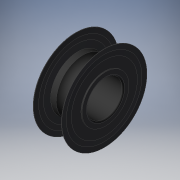
# Autodesk Inventor part: SKF_608-2RSL_PART1
Saved by Autodesk Inventor 2019 (Build 230136000, 136)
## iProperties
Created: 2022-07-08
Part Number: SKF_608-2RSL_PART1
Material: Generic
Catalog Web Link: www.cadenas.de
Description: -Deep groove ball bearings
Vendor: SKF
Document SubType Name: Modeling
Designer: psAdmin
Manufacturer: SKF
Mass: 12 g
Surface Area: 13.7399 cm^2
Volume: 0.419446 cm^3
Density: 1 g/cm^3
Appearance: PSOLRGB-175-175-175
Category: PARTsolutions
Company: SKF
Title: SKF_608-2RSL_PART1
Author: Cadenas PARTsolutions
Comments: Deep groove ball bearings
PSOL_IDENT_0: {$CADENAS_DATA/23d-libs/skf/bearings_units_and_housings/ball_bearings/deep_groove_ball_bearings/bb1_
PSOL_IDENT_1: 001_101.prj},202 {VTYP=3D},{NB=SKF_608-2RSL_PART1},{LINA=SKF_608-2RSL_PART1},{NN=BB1_001_101_PART1},
PSOL_IDENT_2: {NOPRJ=TRUE},{DATE=08.07.2022 10:24:27},{GEOMDATE=04.07.2022 10:54:51},{VERSION=},{LINEID=7700},{WBV
PSOL_IDENT_3: AR=},{WBNUMERIC=}  {NB=SKF_608-2RSL_PART1},{LINA=SKF_608-2RSL_PART1},{KT=DUMMY},{DESIGNATION=608-2RS
PSOL_IDENT_4: L},{R12=0.30},{DD=8.000},{D=22.000},{B=7.000},{C=},{CX=},{CXX=},{CA=0.000},{XXVARIANT=},{XXDESIGN=Si
PSOL_IDENT_5: ngle row},{XXSEALING=Low-friction seal on both sides},{DESIGN=dgbb2rs},{DESIGNIR=dgbb2rs},{VARIANT=}
PSOL_IDENT_6: ,{DD1=12.15},{DD2=10.55},{DD2X=},{DD2A=10.55},{D1=17.60},{D1X=0.00},{D2=19.2},{D2A=19.20},{D3=},{D3X=
PSOL_IDENT_7: },{D3A=0.000},{D4=},{HH=0.000},{BB=0.000},{BBX=},{BBA=0.000},{FF=},{R0MAX=0.000},{R0=0.000},{PITCH=1
PSOL_IDENT_8: 4.70},{DW=3.969},{DDAMIN=10.000},{DDAMAX=10.500},{DDBMIN=0.000},{DDBMAX=0.000},{DBMIN=0.000},{DAMAX=
PSOL_IDENT_9: 20.000},{BBAMIN=0.000},{CAMAX=0.000},{RAMAX=0.300},{LOAD1=3.450},{LOAD2=1.370},{LOAD3=0.057},{SPEED1=
PSOL_IDENT_10: 75000},{SPEED2=38000},{KR=0.025},{F0=12.000},{Z=7},{II=1},{MASS=0.012},{BEARING=608-2RSL},{RING=},{H
PSOL_IDENT_11: ELP=2.200},{HELP2=1.400},{DD1ALG=6.075},{YALG=6.075},{PITCH1=14.700},{DW1=3.969},{YALG1=8.800},{HALG
PSOL_IDENT_12: 1=2.200},{SH=5.275},{CU=0.606},{HALG=2.075},{B1=0},{SHIELDHELP=2},{D4A=0.000},{FFA=0.000},{RS1=},{HE
PSOL_IDENT_13: LP3=0}
NB: SKF_608-2RSL_PART1
NT: Deep groove ball bearings
NBSYN: SKF_$DESIGNATION._PART1
LINA: SKF_608-2RSL_PART1
CATALOG: SKF
DESIGNATION: 608-2RSL
R12: 0.3
DD: 8
D: 22
B: 7
XXDESIGN: Single row
XXSEALING: Low-friction seal on both sides
DD2: 10.55
D2: 19.2
LOAD1: 3.45
LOAD2: 1.37
LOAD3: 0.057
SPEED1: 75000
SPEED2: 38000
BEARING: 608-2RSL
SUPPLIER: SKF
ARTICLENO: SKF_608-2RSL_PART1
BOMINFO: SKF_608-2RSL_PART1
CREATOR: CADENAS GmbH
Autodesk Inventor part; units mm, degrees
ref_plane "YZ Plane" through (0, 0, 0) normal (1, 0, 0) x (0, 1, 0)
ref_plane "XZ Plane" through (0, 0, 0) normal (0, 1, 0) x (-1, 0, 0)
ref_plane "XY Plane" through (0, 0, 0) normal (0, 0, 1) x (1, 0, 0)
sketch "Sketch_58" plane through (0, 0, 0) normal (0, 0, 1) x (1, 0, 0)
  line L0 (50, 0) -> (-50, 0)
  line L1 (0, 5.975) -> (0, 4.3)
  arc A0 (0, 4.3) -> (0.3, 4) centre (0.3, 4.3) ccw
  line L2 (0.3, 4) -> (6.7, 4)
  arc A1 (6.7, 4) -> (7, 4.3) centre (6.7, 4.3) ccw
  line L3 (7, 4.3) -> (7, 5.975)
  arc A2 (7, 5.975) -> (6.9, 6.075) centre (6.9, 5.975) ccw
  line L4 (6.9, 6.075) -> (5.0207, 6.075)
  arc A3 (1.9793, 6.075) -> (5.0207, 6.075) centre (3.5, 7.35) ccw
  line L5 (1.9793, 6.075) -> (0.1, 6.075)
  arc A4 (0.1, 6.075) -> (0, 5.975) centre (0.1, 5.975) ccw
  constraints: 12 end point, 10 point on circle, 5 centre point
revolve "Revolution1" add sketch "Sketch_58" angle 360 about axis through (50, 0, 0) along (1, 0, 0)
sketch "Sketch_59" plane through (0, 0, 0) normal (0, 0, 1) x (1, 0, 0)
  line L0 (50, 0) -> (-50, 0)
  line L1 (0, 8.95) -> (0, 5.275)
  line L2 (0, 5.275) -> (0.4535, 5.275)
  arc A0 (0.4535, 5.275) -> (0.706, 5.5275) centre (0.4535, 5.5275) ccw
  line L3 (0.706, 5.5275) -> (0.706, 8.344)
  line L4 (0.706, 8.344) -> (6.294, 8.344)
  line L5 (6.294, 8.344) -> (6.294, 5.5275)
  arc A1 (6.294, 5.5275) -> (6.5465, 5.275) centre (6.5465, 5.5275) ccw
  line L6 (6.5465, 5.275) -> (7, 5.275)
  line L7 (7, 5.275) -> (7, 8.95)
  line L8 (7, 8.95) -> (0, 8.95)
  constraints: 18 end point, 4 point on circle, 2 centre point
revolve "Revolution2" cut sketch "Sketch_59" angle 360 about axis through (50, 0, 0) along (1, 0, 0)
sketch "Sketch_60" plane through (0, 0, 0) normal (0, 0, 1) x (1, 0, 0)
  line L0 (2, 0) -> (-2, 0)
  line L1 (0.27, 9.6) -> (0.315, 8.5188)
  line L2 (0.315, 8.5188) -> (0.27, 7.4375)
  line L3 (0.27, 7.4375) -> (0.27, 5.275)
  line L4 (0.27, 5.275) -> (0.36, 5.275)
  line L5 (0.36, 5.275) -> (0.45, 7.4375)
  line L6 (0.45, 7.4375) -> (0.45, 8.5188)
  line L7 (0.45, 8.5188) -> (0.36, 9.6)
  line L8 (0.36, 9.6) -> (0.27, 9.6)
  constraints: 18 end point
revolve "Revolution3" add sketch "Sketch_60" angle 360 about axis through (2, 0, 0) along (1, 0, 0)
sketch "Sketch_61" plane through (0, 0, 0) normal (0, 0, 1) x (1, 0, 0)
  line L0 (2, 0) -> (-2, 0)
  line L1 (6.55, 7.4375) -> (6.64, 5.275)
  line L2 (6.64, 5.275) -> (6.73, 5.275)
  line L3 (6.73, 5.275) -> (6.73, 7.4375)
  line L4 (6.73, 7.4375) -> (6.685, 8.5188)
  line L5 (6.685, 8.5188) -> (6.73, 9.6)
  line L6 (6.73, 9.6) -> (6.64, 9.6)
  line L7 (6.64, 9.6) -> (6.55, 8.5188)
  line L8 (6.55, 8.5188) -> (6.55, 7.4375)
  constraints: 18 end point
revolve "Revolution4" add sketch "Sketch_61" angle 360 about axis through (2, 0, 0) along (1, 0, 0)
body "Solid1"
